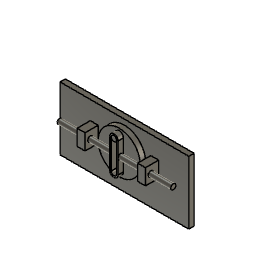
Scotch Yoke Mechanism (Autodesk Fusion 360 design; units mm, degrees)
Autodesk Fusion 360 part; units mm, degrees
sketch "Sketch1" plane through (0, 0, 0) normal (0, 1, 0) x (1, 0, 0)
  line L0 (122.5, -60) -> (-122.5, -60)
  line L1 (-122.5, -60) -> (-122.5, 60)
  line L2 (-122.5, 60) -> (122.5, 60)
  line L3 (122.5, 60) -> (122.5, -60)
  line L4 (122.5, -60) -> (-122.5, 60) construction
  line L5 (-122.5, -60) -> (122.5, 60) construction
  line L6 (-50, -25) -> (-65, -25)
  line L7 (-65, -25) -> (-65, 5)
  line L8 (-65, 5) -> (-50, 5)
  line L9 (-50, 5) -> (-50, -25)
  line L10 (-50, -25) -> (-65, 5) construction
  line L11 (-65, -25) -> (-50, 5) construction
  line L12 (65, -25) -> (50, -25)
  line L13 (50, -25) -> (50, 5)
  line L14 (50, 5) -> (65, 5)
  line L15 (65, 5) -> (65, -25)
  line L16 (65, -25) -> (50, 5) construction
  line L17 (50, -25) -> (65, 5) construction
  circle A0 centre (0, -10) radius 10.5
  point P0 (-57.5, -10)
  point P1 (57.5, -10)
  dimension "d1" = 245
  dimension "d2" = 120
  dimension "d3" = 15
  dimension "d4" = 30
  dimension "d5" = 15
  dimension "d6" = 30
  dimension "d7" = 55
  dimension "d8" = 30
  dimension "d9" = 100
  dimension "d10" = 50
  dimension "d11" = 21
  dimension "d12" = 21
  dimension "d13" = 10
  constraint horizontal L0
  constraint perpendicular L0 L1
  constraint parallel L0 L2
  constraint parallel L1 L3
  constraint coincident L4 origin
  constraint coincident L5 origin
  constraint horizontal L6
  constraint perpendicular L6 L7
  constraint parallel L6 L8
  constraint parallel L7 L9
  constraint coincident L10 P0
  constraint coincident L11 P0
  constraint horizontal L12
  constraint perpendicular L12 L13
  constraint parallel L12 L14
  constraint parallel L13 L15
  constraint coincident L16 P1
  constraint coincident L17 P1
  constraint vertical origin A0.centre
  measures "d1" distance of L1.end L2.end
  measures "d2" distance of L0.end L1.end
  measures "d3" distance of L7.end L8.end
  measures "d4" distance of L6.end L7.end
  measures "d5" distance of L13.end L14.end
  measures "d6" distance of L12.end L13.end
  measures "d7" distance of L2 L8
  measures "d8" distance of L8 L12
  measures "d9" distance of L9 L13
  measures "d10" distance of origin L9
  measures "d11" diameter of A0
  measures "d12" diameter of A0
  measures "d13" distance of origin A0.centre
extrude "Extrude1" add sketch "Sketch1" along normal blind 10 makes body 1
extrude "Extrude2" add sketch "Sketch1" along normal blind 10 and the other way blind 25 contours L6 L7 L8 L9 | L12 L13 L14 L15 bodies 1
sketch "Sketch2" plane through (-65, 0, 0) normal (-1, 0, 0) x (0, -1, 0)
  line L0 (0, 25) -> (0, -5)
  line L1 (0, -5) -> (25, -5)
  line L2 (25, -5) -> (25, 25)
  line L3 (25, 25) -> (0, 25)
  circle A0 centre (15, 10) radius 5
  line L4 (0, 60) -> (0, -60)
  dimension "d20" = 10
  dimension "d21" = 15
  dimension "d22" = 15
  measures "d20" diameter of A0
  measures "d21" distance of L1 A0.centre
  measures "d22" distance of A0.centre L4
extrude "Extrude3" cut sketch "Sketch2" against normal through all contours A0 bodies 1
copy_body "Body->Comp1" bodies 1 removing the originals makes body 2 in component "Base"
sketch "Sketch3" plane through (0, 0, 0) normal (0, 1, 0) x (1, 0, 0)
  line L0 (144.9958, -110.0049) -> (144.9958, -166.0049)
  line L1 (154.9958, -110.0049) -> (154.9958, -166.0049)
  arc A0 (144.9958, -166.0049) -> (154.9958, -166.0049) centre (149.9958, -166.0049) ccw
  arc A1 (154.9958, -110.0049) -> (144.9958, -110.0049) centre (149.9958, -110.0049) ccw
  arc A2 (141.9958, -166.0049) -> (157.9958, -166.0049) centre (149.9958, -166.0049) ccw
  line L2 (157.9958, -110.0049) -> (157.9958, -166.0049)
  arc A3 (157.9958, -110.0049) -> (141.9958, -110.0049) centre (149.9958, -110.0049) ccw
  line L3 (141.9958, -110.0049) -> (141.9958, -166.0049)
  dimension "d24" = 10
  dimension "d25" = 10
  dimension "d26" = 56
  dimension "d27" = -3
  constraint tangent L0 A0
  constraint tangent L1 A0
  constraint tangent L0 A1
  constraint tangent L1 A1
  constraint parallel L0 L1
  constraint vertical A0.centre A1.centre
  measures "d24" diameter of A0
  measures "d25" diameter of A1
  measures "d26" vertical distance of A0.centre A1.centre
extrude "Extrude4" add sketch "Sketch3" along normal blind 10 separate body makes body 3
sketch "Sketch4" plane through (157.9958, 0, 0) normal (1, 0, 0) x (0, 1, 0)
  line L0 (0, 166.0049) -> (0, 110.0049)
  line L1 (0, 110.0049) -> (10, 110.0049)
  line L2 (10, 110.0049) -> (10, 166.0049)
  line L3 (10, 166.0049) -> (0, 166.0049)
  circle A0 centre (5, 138.0049) radius 5
  dimension "d30" = 10
  dimension "d31" = 28
  dimension "d32" = 5
  measures "d30" diameter of A0
  measures "d31" distance of L3 A0.centre
  measures "d32" distance of L2 A0.centre
extrude "Extrude5" add sketch "Sketch4" along normal blind 100 contours A0 bodies 3
ref_plane "WorkPlane1" through (149.9958, 5, 138.0049) normal (1, 0, 0) x (0, 0, -1)
mirror "Mirror1" about plane through (149.9958, 5, 138.0049) normal (1, 0, 0) of "Extrude5"
copy_body "Body->Comp2" bodies 3 removing the originals makes body 4 in component "Sliding Pair"
sketch "Sketch5" plane through (0, 0, 0) normal (0, 1, 0) x (1, 0, 0)
  circle A0 centre (-192.7727, -130.3001) radius 40
  dimension "d37" = 80
  measures "d37" diameter of A0
extrude "Extrude6" add sketch "Sketch5" along normal blind 10 separate body makes body 5
sketch "Sketch6" plane through (0, 0, 0) normal (0, -1, 0) x (1, 0, 0)
  circle A0 centre (-192.7727, 130.3001) radius 40
  circle A1 centre (-192.7727, 158.3001) radius 5
  dimension "d40" = 10
  dimension "d41" = 28
  constraint vertical A0.centre A1.centre
  measures "d40" diameter of A1
  measures "d41" vertical distance of A0.centre A1.centre
extrude "Extrude7" add sketch "Sketch6" along normal blind 10 contours A1 bodies 5
sketch "Sketch7" plane through (0, 10, 0) normal (0, 1, 0) x (-1, 0, 0)
  circle A0 centre (192.7727, 130.3001) radius 40
  circle A1 centre (192.7727, 130.3001) radius 10
  dimension "d44" = 20
  constraint concentric A0 A1
  measures "d44" diameter of A1
extrude "Extrude8" add sketch "Sketch7" along normal blind 10 contours A1 bodies 5
copy_body "Body->Comp3" bodies 5 removing the originals makes body 6 in component "Component"
component "Base" placed x (1, 0, 0) y (0, 1, 0) z (0, 0, 1) at (0, 0, 0)
component "Sliding Pair" placed x (1, 0, 0) y (0, 1, 0) z (0, 0, 1) at (-149.9958, -20, -128.0049)
component "Component" placed x (1, 0, 0) y (0, 1, 0) z (0, 0, 1) at (192.7727, -10, -120.3001)
equation "d7 = 120 mm - 35 mm - 30 mm"
